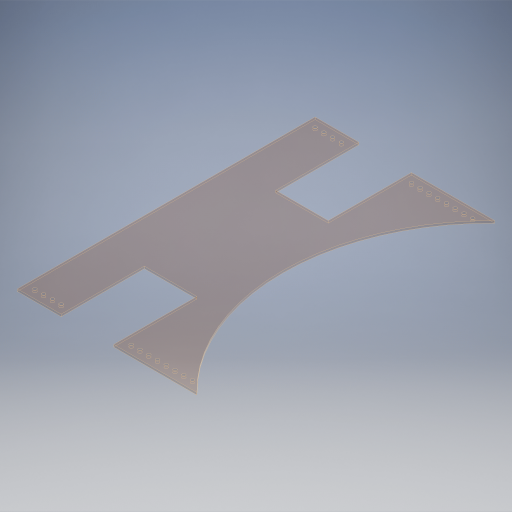
# Autodesk Inventor part: Polycarbonate-Note-Intakaur-Cover
Saved by Autodesk Inventor 2024.2 (Build 282272000, 272)
## iProperties
Created: 2024-02-11
Part Number: Polycarbonate-Note-Intakaur-Cover
Material: Polycarbonate, Smoke
Document SubType Name: Modeling
Designer: rohan
Density: 1.2 g/cm^3
Appearance: Polycarbonate - Smoked
Author: rohan
Autodesk Inventor part; units mm, degrees
ref_plane "YZ Plane" through (0, 0, 0) normal (1, 0, 0) x (0, 1, 0)
ref_plane "XZ Plane" through (0, 0, 0) normal (0, 1, 0) x (-1, 0, 0)
ref_plane "XY Plane" through (0, 0, 0) normal (0, 0, 1) x (1, 0, 0)
sketch "Sketch1" plane through (0, 0, 0) normal (0, 1, 0) x (-1, 0, 0)
  arc A0 (210.5939, -215.9) -> (210.5939, 215.9) centre (0, 0) ccw
  line L0 (470.9439, 215.9) -> (470.9439, -215.9)
  line L1 (470.9439, 215.9) -> (407.4439, 215.9)
  line L2 (407.4439, 215.9) -> (407.4439, 95.25)
  line L3 (407.4439, 95.25) -> (331.2439, 95.25)
  line L4 (331.2439, 95.25) -> (331.2439, 215.9)
  line L5 (470.9439, -215.9) -> (407.4439, -215.9)
  line L6 (407.4439, -215.9) -> (407.4439, -95.25)
  line L7 (407.4439, -95.25) -> (331.2439, -95.25)
  line L8 (331.2439, -95.25) -> (331.2439, -215.9)
  line L9 (331.2439, 215.9) -> (210.5939, 215.9)
  line L10 (331.2439, -215.9) -> (210.5939, -215.9)
  circle A1 centre (458.2439, 203.2) radius 2.4892
  circle A2 centre (445.5439, 203.2) radius 2.4892
  circle A3 centre (432.8439, 203.2) radius 2.4892
  circle A4 centre (420.1439, 203.2) radius 2.4892
  circle A5 centre (318.5439, 203.2) radius 2.4892
  circle A6 centre (305.8439, 203.2) radius 2.4892
  circle A7 centre (293.1439, 203.2) radius 2.4892
  circle A8 centre (280.4439, 203.2) radius 2.4892
  circle A9 centre (267.7439, 203.2) radius 2.4892
  circle A10 centre (255.0439, 203.2) radius 2.4892
  circle A11 centre (242.3439, 203.2) radius 2.4892
  circle A12 centre (229.6439, 203.2) radius 2.4892
  line L11 (597.6164, 0) -> (168.2721, 0) construction
  circle A13 centre (458.2439, -203.2) radius 2.4892
  circle A14 centre (445.5439, -203.2) radius 2.4892
  circle A15 centre (432.8439, -203.2) radius 2.4892
  circle A16 centre (420.1439, -203.2) radius 2.4892
  circle A17 centre (318.5439, -203.2) radius 2.4892
  circle A18 centre (305.8439, -203.2) radius 2.4892
  circle A19 centre (293.1439, -203.2) radius 2.4892
  circle A20 centre (280.4439, -203.2) radius 2.4892
  circle A21 centre (267.7439, -203.2) radius 2.4892
  circle A22 centre (255.0439, -203.2) radius 2.4892
  circle A23 centre (242.3439, -203.2) radius 2.4892
  circle A24 centre (229.6439, -203.2) radius 2.4892
  dimension "d0" = 603.2002
  dimension "d1" = 431.8
  dimension "d2" = 63.5
  dimension "d3" = 120.65
  dimension "d4" = 76.2
  dimension "d5" = 63.5
  dimension "d6" = 120.65
  dimension "d7" = 76.2
  dimension "d8" = 120.65
  dimension "d9" = 120.65
  dimension "d10" = 4.9784
  dimension "d11" = 12.7
  dimension "d12" = 12.7
  dimension "d15" = 12.7
  dimension "d20" = 4.9784
  dimension "d21" = 12.7
  dimension "d22" = 12.7
  dimension "d25" = 12.7
  dimension "d30" = 12.7
  constraints: 25 centre point, 24 end point, 12 symmetric about line, 8 horizontal, 4 perpendicular, 2 point on circle, 2 vertical, 1 coincident, 1 point on line, 32 other
  measures "d0" diameter of A0
  measures "d1" distance of L0.start L0.end
  measures "d2" distance of L0.start L1.end
  measures "d3" distance of L1.end L2.end
  measures "d4" distance of L2.end L3.end
  measures "d5" distance of L0.end L5.end
  measures "d6" distance of L5.end L6.end
  measures "d7" distance of L6.end L7.end
  measures "d8" distance of L4.end L9.end
  measures "d9" distance of L8.end L10.end
  measures "d10" diameter of A1
  measures "d11" distance from line of L0 A1.centre
  measures "d12" distance from line of L1 A1.centre
  measures "d15" distance of A1.centre A2.centre
  measures "d20" diameter of A5
  measures "d21" distance from line of L4 A5.centre
  measures "d22" distance from line of L9 A5.centre
  measures "d25" distance of A5.centre A6.centre
  measures "d30" distance from line of L5 A13.centre
extrude "Extrusion1" add sketch "Sketch1" along normal blind 6.35
sketch "Sketch2" plane through (0, 6.35, 0) normal (0, 1, 0) x (1, 0, 0)
  line L0 (-407.4439, -215.9) -> (-407.4439, -95.25) projected
  line L1 (-407.4439, -95.25) -> (-331.2439, -95.25) projected
  line L2 (-331.2439, -95.25) -> (-331.2439, -215.9) projected
  line L3 (-331.2439, -215.9) -> (-210.5939, -215.9) projected
  arc A0 (-210.5939, 215.9) -> (-210.5939, -215.9) centre (0, 0) ccw projected
  line L4 (-210.5939, 215.9) -> (-331.2439, 215.9) projected
  line L5 (-331.2439, 215.9) -> (-331.2439, 95.25) projected
  line L6 (-331.2439, 95.25) -> (-407.4439, 95.25) projected
  line L7 (-407.4439, 95.25) -> (-407.4439, 215.9) projected
  line L8 (-407.4439, 215.9) -> (-470.9439, 215.9) projected
  line L9 (-470.9439, 215.9) -> (-470.9439, -215.9) projected
  line L10 (-470.9439, -215.9) -> (-407.4439, -215.9) projected
  circle A1 centre (-305.8439, 203.2) radius 2.4892 projected
  circle A2 centre (-458.2439, 203.2) radius 2.4892 projected
  circle A3 centre (-432.8439, 203.2) radius 2.4892 projected
  circle A4 centre (-420.1439, 203.2) radius 2.4892 projected
  circle A5 centre (-305.8439, -203.2) radius 2.4892 projected
  circle A6 centre (-318.5439, -203.2) radius 2.4892 projected
  circle A7 centre (-420.1439, -203.2) radius 2.4892 projected
  circle A8 centre (-432.8439, -203.2) radius 2.4892 projected
  circle A9 centre (-445.5439, -203.2) radius 2.4892 projected
  circle A10 centre (-458.2439, -203.2) radius 2.4892 projected
  circle A11 centre (-445.5439, 203.2) radius 2.4892 projected
  circle A12 centre (-318.5439, 203.2) radius 2.4892 projected
  circle A13 centre (-293.1439, 203.2) radius 2.4892 projected
  circle A14 centre (-280.4439, 203.2) radius 2.4892 projected
  circle A15 centre (-267.7439, 203.2) radius 2.4892 projected
  circle A16 centre (-255.0439, 203.2) radius 2.4892 projected
  circle A17 centre (-242.3439, 203.2) radius 2.4892 projected
  circle A18 centre (-229.6439, 203.2) radius 2.4892 projected
  circle A19 centre (-229.6439, -203.2) radius 2.4892 projected
  circle A20 centre (-242.3439, -203.2) radius 2.4892 projected
  circle A21 centre (-255.0439, -203.2) radius 2.4892 projected
  circle A22 centre (-267.7439, -203.2) radius 2.4892 projected
  circle A23 centre (-280.4439, -203.2) radius 2.4892 projected
  circle A24 centre (-293.1439, -203.2) radius 2.4892 projected
extrude "Extrusion2" cut sketch "Sketch2" against normal blind 3.175
body "Solid1"
